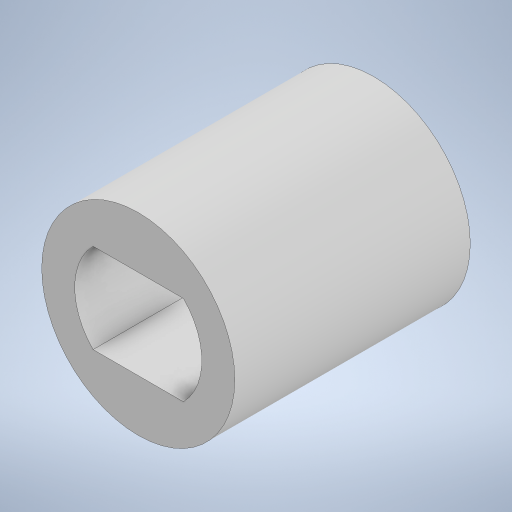
# Autodesk Inventor part: bağlantı elemanı
Saved by Autodesk Inventor 2023.2 (Build 272271000, 271)
## iProperties
Created: 2022-11-25
Part Number: bağlantı elemanı
Material: Generic
Document SubType Name: Modeling
Designer: omrfrkmll
Density: 1 g/cm^3
Appearance: Default
Author: omrfrkmll
Autodesk Inventor part; units mm, degrees
ref_plane "YZ Plane" through (0, 0, 0) normal (1, 0, 0) x (0, 1, 0)
ref_plane "XZ Plane" through (0, 0, 0) normal (0, 1, 0) x (-1, 0, 0)
ref_plane "XY Plane" through (0, 0, 0) normal (0, 0, 1) x (1, 0, 0)
sketch "Sketch1" plane through (0, 0, 0) normal (0, 0, 1) x (1, 0, 0)
  line L0 (-1.9183, 1.9) -> (1.9183, 1.9)
  line L1 (-3.0684, 0) -> (3.272, 0)
  line L2 (-1.9183, -1.9) -> (1.9183, -1.9)
  circle A0 centre (0, 0) radius 4.1
  arc A1 (-1.9183, 1.9) -> (-1.9183, -1.9) centre (0, 0) ccw
  arc A2 (1.9183, -1.9) -> (1.9183, 1.9) centre (0, 0) ccw
  dimension "d2" = 3.8
  dimension "d4" = 2.7
  dimension "d5" = 2.7
  constraints: 6 end point, 4 horizontal, 4 point on circle, 3 centre point, 1 coincident, 1 other
  measures "d2" distance between parallel lines of L2 L0
  measures "d4" radius of A2
  measures "d5" radius of A1
extrude "Extrusion1" add sketch "Sketch1" along normal blind 10
body "Solid1"
